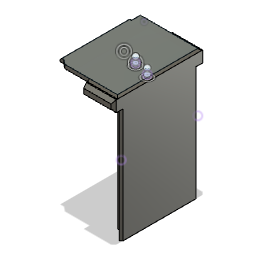
LID (Autodesk Fusion 360 design; units mm, degrees)
Autodesk Fusion 360 part; units mm, degrees
(part 1 of 2)
sketch "Sketch1" plane through (0, 0, 0) normal (0, 1, 0) x (1, 0, 0)
  line L0 (0, 0) -> (18.5, 0)
  line L1 (18.5, 0) -> (18.5, -27.5)
  line L2 (18.5, -27.5) -> (0, -27.5)
  line L3 (0, -27.5) -> (0, 0)
  circle A0 centre (18.5, 0) radius 0.625
  circle A1 centre (0, 0) radius 0.625
  circle A2 centre (0, -27.5) radius 0.625
  circle A3 centre (18.5, -27.5) radius 0.625
  line L4 (-2, -29.5) -> (-2, 2)
  line L5 (-2, 2) -> (20.5, 2)
  line L6 (20.5, 2) -> (20.5, -29.5)
  line L7 (20.5, -29.5) -> (-2, -29.5)
  dimension "d1" = 18.5
  dimension "d2" = 27.5
  dimension "d3" = 1.25
  dimension "d4" = 1.25
  dimension "d5" = 1.25
  dimension "d6" = 1.25
  dimension "d7" = -2
  constraint horizontal L0
  constraint vertical L1
  constraint horizontal L2
  constraint vertical L3
  constraint coincident L0.start L3.end
  constraint coincident L0.end L1.start
  constraint coincident L2.end L3.start
  constraint coincident L1.end L2.start
  measures "d1" distance of L0.start L0.end
  measures "d2" distance of L0.start L2.end
  measures "d3" diameter of A0
  measures "d4" diameter of A1
  measures "d5" diameter of A2
  measures "d6" diameter of A3
sketch "Sketch2" plane through (0, 0, 0) normal (0, -1, 0) x (1, 0, 0)
  circle A0 centre (18.5, 27.5) radius 0.625
  circle A1 centre (18.5, 0) radius 0.625
  circle A2 centre (0, 27.5) radius 0.625
  circle A3 centre (0, 0) radius 0.625
  line L0 (20.5, -2) -> (20.5, 29.5)
  line L1 (20.5, 29.5) -> (-2, 29.5)
  line L2 (-2, 29.5) -> (-2, -2)
  line L3 (-2, -2) -> (20.5, -2)
  line L4 (20.5, 29.5) -> (9.25, 29.5)
  line L5 (9.25, 29.5) -> (9.25, 13.75)
  line L6 (9.25, 13.75) -> (20.5, 13.75)
  line L7 (20.5, 13.75) -> (20.5, 29.5)
  circle A4 centre (9.25, 13.75) radius 4.3
  dimension "d10" = 11.25
  dimension "d11" = 15.75
  dimension "d12" = 8.6
  constraint horizontal L4
  constraint vertical L5
  constraint horizontal L6
  constraint vertical L7
  constraint coincident L0.end L1.start
  constraint coincident L5.end L6.start
  measures "d10" distance of L0.end L4.end
  measures "d11" distance of L0.end L6.end
  measures "d12" diameter of A4
sketch "Sketch3" plane through (0, 3, 0) normal (0, 1, 0) x (-1, 0, 0)
  circle A0 centre (-9.25, 13.75) radius 4.3
  circle A1 centre (-18.5, 27.5) radius 0.625
  circle A2 centre (-18.5, 0) radius 0.625
  circle A3 centre (0, 27.5) radius 0.625
  circle A4 centre (0, 0) radius 0.625
  line L0 (-20.5, 29.5) -> (-20.5, -2)
  line L1 (-20.5, -2) -> (2, -2)
  line L2 (2, -2) -> (2, 29.5)
  line L3 (2, 29.5) -> (-20.5, 29.5)
  line L4 (-15.4346, 2.2358) -> (-15.4346, 25.68) construction
  line L5 (-15.4346, 25.68) -> (-19.6447, 25.68) construction
  line L6 (-19.6447, 25.68) -> (-19.6447, 2.2358) construction
  line L7 (-19.6447, 2.2358) -> (-15.4346, 2.2358) construction
  line L8 (-1.4263, -7.8741) -> (1.1046, 16.1483) construction
  line L9 (1.1046, 16.1483) -> (-2.8567, 16.5657) construction
  line L10 (-2.8567, 16.5657) -> (-5.3876, -7.4567) construction
  line L11 (-5.3876, -7.4567) -> (-1.4263, -7.8741) construction
sketch "Sketch4" plane through (0, 0, 0) normal (0, 1, 0) x (1, 0, 0)
  line L0 (0, 0) -> (122.2, 0)
  line L1 (122.2, 0) -> (122.2, -193)
  line L2 (122.2, -193) -> (0, -193)
  line L3 (0, -193) -> (0, 0)
  dimension "d17" = 122.2
  dimension "d18" = 193
  constraint horizontal L0
  constraint vertical L1
  constraint horizontal L2
  constraint vertical L3
  constraint coincident L0.start L3.end
  measures "d17" distance of L0.start L0.end
  measures "d18" distance of L0.start L2.end
extrude "Extrude4" add sketch "Sketch4" along normal blind 5 makes body 1
extrude "Extrude5" cut 1 faces at (40.7333, 5, 64.3333) along direction (0, -1, 0) blind 5 on bodies 1 bodies 1
sketch "Sketch5" plane through (0, 0, 0) normal (0, 1, 0) x (1, 0, 0)
  line L0 (0, 0) -> (122.2, 0)
  line L1 (122.2, 0) -> (122.2, -193)
  line L2 (122.2, -193) -> (0, -193)
  line L3 (0, -193) -> (0, 0)
  dimension "d23" = 122.2
  dimension "d24" = 193
  constraint horizontal L0
  constraint vertical L1
  constraint horizontal L2
  constraint vertical L3
  constraint coincident L0.start L3.end
  measures "d23" distance of L0.start L0.end
  measures "d24" distance of L0.start L2.end
extrude "Extrude6" add sketch "Sketch5" along normal blind 5 bodies 1
sketch "Sketch6" plane through (0, 5, 0) normal (0, 1, 0) x (-1, 0, 0)
  line L0 (0, 193) -> (-122.2, 193)
  line L1 (-122.2, 193) -> (-122.2, 0)
  line L2 (-122.2, 0) -> (0, 0)
  line L3 (0, 0) -> (0, 193)
  line L4 (0, 193) -> (-10, 193)
  line L5 (-10, 193) -> (-10, 158)
  line L6 (-10, 158) -> (0, 158)
  line L7 (0, 158) -> (0, 193)
  line L8 (0, 0) -> (-10, 0)
  line L9 (-10, 0) -> (-10, 35)
  line L10 (-10, 35) -> (0, 35)
  line L11 (0, 35) -> (0, 0)
  line L12 (-10, 158) -> (-60, 158)
  line L13 (-60, 158) -> (-60, 35)
  line L14 (-60, 35) -> (-10, 35)
  line L15 (-10, 35) -> (-10, 158)
  dimension "d27" = 10
  dimension "d28" = 35
  dimension "d29" = 10
  dimension "d30" = 35
  dimension "d31" = 50
  constraint horizontal L4
  constraint vertical L5
  constraint horizontal L6
  constraint vertical L7
  constraint coincident L0.start L3.end
  constraint horizontal L8
  constraint vertical L9
  constraint horizontal L10
  constraint vertical L11
  constraint coincident L2.end L3.start
  constraint horizontal L12
  constraint vertical L13
  constraint horizontal L14
  constraint vertical L15
  measures "d27" distance of L0.start L4.end
  measures "d28" distance of L0.start L6.end
  measures "d29" distance of L2.end L8.end
  measures "d30" distance of L2.end L10.end
  measures "d31" distance of L5.end L12.end
extrude "Extrude7" cut sketch "Sketch6" against normal blind 5 contours L12 L13 L14 L15 bodies 1
sketch "Sketch7" plane through (0, 5, 0) normal (0, 1, 0) x (-1, 0, 0)
  line L0 (-60, 158) -> (-10, 158)
  line L1 (-10, 158) -> (-10, 35)
  line L2 (-10, 35) -> (-60, 35)
  line L3 (-60, 35) -> (-60, 158)
  line L4 (0, 193) -> (-122.2, 193)
  line L5 (-122.2, 193) -> (-122.2, 0)
  line L6 (-122.2, 0) -> (0, 0)
  line L7 (0, 0) -> (0, 193)
  line L8 (-122.2, 193) -> (-105.075, 193)
  line L9 (-105.075, 193) -> (-105.075, 102)
  line L10 (-105.075, 102) -> (-122.2, 102)
  line L11 (-122.2, 102) -> (-122.2, 193)
  circle A0 centre (-105.075, 102) radius 4
  dimension "d34" = 17.125
  dimension "d35" = 91
  dimension "d36" = 8
  constraint horizontal L8
  constraint vertical L9
  constraint horizontal L10
  constraint vertical L11
  constraint coincident L4.end L5.start
  constraint coincident L9.end L10.start
  measures "d34" distance of L4.end L8.end
  measures "d35" distance of L4.end L10.end
  measures "d36" diameter of A0
extrude "Extrude8" cut sketch "Sketch7" against normal blind 5 contours L9 L10 A0 | L9 L10 A0 bodies 1
sketch "Sketch8" plane through (0, 5, 0) normal (0, 1, 0) x (-1, 0, 0)
  circle A0 centre (-105.075, 102) radius 4
  line L0 (-60, 158) -> (-10, 158)
  line L1 (-10, 158) -> (-10, 35)
  line L2 (-10, 35) -> (-60, 35)
  line L3 (-60, 35) -> (-60, 158)
  line L4 (0, 193) -> (-122.2, 193)
  line L5 (-122.2, 193) -> (-122.2, 0)
  line L6 (-122.2, 0) -> (0, 0)
  line L7 (0, 0) -> (0, 193)
  line L8 (-105.075, 102) -> (-63.325, 102)
  line L9 (-63.325, 102) -> (-63.325, 91)
  line L10 (-63.325, 91) -> (-105.075, 91)
  line L11 (-105.075, 91) -> (-105.075, 102)
  line L12 (-60, 158, -5) -> (-52, 158, -5)
  line L13 (-52, 158, -5) -> (-52, 35, -5)
  line L14 (-52, 35, -5) -> (-60, 35, -5)
  line L15 (-60, 35, -5) -> (-60, 158, -5)
  circle A1 centre (-63.325, 91) radius 4
  point P0 (-60, 158)
  dimension "d39" = 41.75
  dimension "d40" = 11
  dimension "d41" = 8
  dimension "d42" = 8
  constraint horizontal L8
  constraint vertical L9
  constraint horizontal L10
  constraint vertical L11
  constraint coincident A0.centre L8.start
  constraint coincident P0 L0.start
  constraint coincident L9.end L10.start
  measures "d39" distance of A0.centre L8.end
  measures "d40" distance of A0.centre L10.end
  measures "d42" diameter of A1
extrude "Extrude9" add sketch "Sketch8" along normal blind 5 contours L12 L13 L14 L15 in plane through (0, 0, 0) normal (0, 1, 0) bodies 1
sketch "Sketch9" plane through (0, 5, 0) normal (0, 1, 0) x (-1, 0, 0)
  circle A0 centre (-105.075, 102) radius 4
  line L0 (-52, 158) -> (-10, 158)
  line L1 (-10, 158) -> (-10, 35)
  line L2 (-10, 35) -> (-52, 35)
  line L3 (-52, 35) -> (-52, 158)
  line L4 (0, 193) -> (-122.2, 193)
  line L5 (-122.2, 193) -> (-122.2, 0)
  line L6 (-122.2, 0) -> (0, 0)
  line L7 (0, 0) -> (0, 193)
  line L8 (-105.075, 102) -> (-63.325, 102)
  line L9 (-63.325, 102) -> (-63.325, 91)
  line L10 (-63.325, 91) -> (-105.075, 91)
  line L11 (-105.075, 91) -> (-105.075, 102)
  circle A1 centre (-63.325, 91) radius 4
  dimension "d45" = 41.75
  dimension "d46" = 11
  dimension "d47" = 8
  constraint horizontal L8
  constraint vertical L9
  constraint horizontal L10
  constraint vertical L11
  constraint coincident A0.centre L8.start
  constraint coincident L9.end L10.start
  measures "d45" distance of A0.centre L8.end
  measures "d46" distance of A0.centre L10.end
  measures "d47" diameter of A1
extrude "Extrude10" cut sketch "Sketch9" against normal blind 5 contours L9 L10 A1 | L9 L10 A1 bodies 1
sketch "Sketch10" plane through (0, 5, 0) normal (0, 1, 0) x (-1, 0, 0)
  circle A0 centre (-63.325, 91) radius 4
  circle A1 centre (-105.075, 102) radius 4
  line L0 (-52, 158) -> (-10, 158)
  line L1 (-10, 158) -> (-10, 35)
  line L2 (-10, 35) -> (-52, 35)
  line L3 (-52, 35) -> (-52, 158)
  line L4 (0, 193) -> (-122.2, 193)
  line L5 (-122.2, 193) -> (-122.2, 0)
  line L6 (-122.2, 0) -> (0, 0)
  line L7 (0, 0) -> (0, 193)
  line L8 (-122.2, 0) -> (-117.2, 0)
  line L9 (-117.2, 0) -> (-117.2, 2)
  line L10 (-117.2, 2) -> (-122.2, 2)
  line L11 (-122.2, 2) -> (-122.2, 0)
  line L12 (-117.2, 2) -> (-31.2, 2)
  line L13 (-31.2, 2) -> (-31.2, 26)
  line L14 (-31.2, 26) -> (-117.2, 26)
  line L15 (-117.2, 26) -> (-117.2, 2)
  dimension "d50" = 5
  dimension "d51" = 2
  dimension "d52" = 86
  dimension "d53" = 24
  constraint horizontal L8
  constraint vertical L9
  constraint horizontal L10
  constraint vertical L11
  constraint coincident L5.end L6.start
  constraint horizontal L12
  constraint vertical L13
  constraint horizontal L14
  constraint vertical L15
  measures "d50" distance of L5.end L8.end
  measures "d51" distance of L5.end L10.end
  measures "d52" distance of L9.end L12.end
  measures "d53" distance of L9.end L14.end
extrude "Extrude11" cut sketch "Sketch10" against normal blind 5 contours L12 L13 L14 L15 bodies 1
sketch "Sketch11" plane through (0, 5, 0) normal (0, 1, 0) x (-1, 0, 0)
  line L0 (-31.2, 2) -> (-117.2, 2)
  line L1 (-117.2, 2) -> (-117.2, 26)
  line L2 (-117.2, 26) -> (-31.2, 26)
  line L3 (-31.2, 26) -> (-31.2, 2)
  circle A0 centre (-63.325, 91) radius 4
  circle A1 centre (-105.075, 102) radius 4
  line L4 (-52, 158) -> (-10, 158)
  line L5 (-10, 158) -> (-10, 35)
  line L6 (-10, 35) -> (-52, 35)
  line L7 (-52, 35) -> (-52, 158)
  line L8 (0, 193) -> (-122.2, 193)
  line L9 (-122.2, 193) -> (-122.2, 0)
  line L10 (-122.2, 0) -> (0, 0)
  line L11 (0, 0) -> (0, 193)
  line L12 (-122.2, 0) -> (5, 0)
  line L13 (5, 0) -> (5, -5)
  line L14 (5, -5) -> (-122.2, -5)
  line L15 (-122.2, -5) -> (-122.2, 0)
  line L16 (-122.2, 193) -> (5, 193)
  line L17 (5, 193) -> (5, 198)
  line L18 (5, 198) -> (-122.2, 198)
  line L19 (-122.2, 198) -> (-122.2, 193)
  line L20 (5, 193) -> (0, 193)
  line L21 (0, 193) -> (0, 0)
  line L22 (0, 0) -> (5, 0)
  line L23 (5, 0) -> (5, 193)
  dimension "d56" = 127.2
  dimension "d57" = 5
  dimension "d58" = 127.2
  dimension "d59" = 5
  constraint horizontal L12
  constraint vertical L13
  constraint horizontal L14
  constraint vertical L15
  constraint coincident L9.end L10.start
  constraint horizontal L16
  constraint vertical L17
  constraint horizontal L18
  constraint vertical L19
  constraint coincident L8.end L9.start
  constraint horizontal L20
  constraint vertical L21
  constraint horizontal L22
  constraint vertical L23
  constraint coincident L10.end L11.start
  measures "d56" distance of L9.end L12.end
  measures "d57" distance of L9.end L14.end
  measures "d58" distance of L8.end L16.end
  measures "d59" distance of L8.end L18.end
extrude "Extrude12" add sketch "Sketch11" along normal blind 5 bodies 1
sketch "Sketch12" plane through (0, 10, 0) normal (0, 1, 0) x (-1, 0, 0)
  line L0 (-117.2, 26) -> (-31.2, 26)
  line L1 (-31.2, 26) -> (-31.2, 2)
  line L2 (-31.2, 2) -> (-117.2, 2)
  line L3 (-117.2, 2) -> (-117.2, 26)
  circle A0 centre (-105.075, 102) radius 4
  line L4 (-10, 35) -> (-52, 35)
  line L5 (-52, 35) -> (-52, 158)
  line L6 (-52, 158) -> (-10, 158)
  line L7 (-10, 158) -> (-10, 35)
  circle A1 centre (-63.325, 91) radius 4
  line L8 (5, -5) -> (5, 198)
  line L9 (5, 198) -> (-122.2, 198)
  line L10 (-122.2, 198) -> (-122.2, -5)
  line L11 (-122.2, -5) -> (5, -5)
  line L12 (5, 198) -> (10, 198)
  line L13 (10, 198) -> (10, -5)
  line L14 (10, -5) -> (5, -5)
  line L15 (5, -5) -> (5, 198)
  dimension "d62" = 5
  constraint horizontal L12
  constraint vertical L13
  constraint horizontal L14
  constraint vertical L15
  constraint coincident L8.end L9.start
  measures "d62" distance of L8.end L12.end
extrude "Extrude13" add sketch "Sketch12" against normal blind 10 contours L8 L12 L13 L14 L15 bodies 1
extrude "Extrude14" add 1 faces at (-6.6667, 0, 130.3333) along direction (0, -1, 0) blind 45 on bodies 1 bodies 1
extrude "Extrude15" cut 1 faces at (-6.6667, -45, 130.3333) along direction (0, 1, 0) blind 5 on bodies 1 bodies 1
sketch "Sketch13" plane through (0, 10, 0) normal (0, 1, 0) x (-1, 0, 0)
  line L0 (-117.2, 26) -> (-31.2, 26)
  line L1 (-31.2, 26) -> (-31.2, 2)
  line L2 (-31.2, 2) -> (-117.2, 2)
  line L3 (-117.2, 2) -> (-117.2, 26)
  circle A0 centre (-105.075, 102) radius 4
  line L4 (-10, 35) -> (-52, 35)
  line L5 (-52, 35) -> (-52, 158)
  line L6 (-52, 158) -> (-10, 158)
  line L7 (-10, 158) -> (-10, 35)
  circle A1 centre (-63.325, 91) radius 4
  line L8 (10, 198) -> (-122.2, 198)
  line L9 (-122.2, 198) -> (-122.2, -5)
  line L10 (-122.2, -5) -> (10, -5)
  line L11 (10, -5) -> (10, 198)
  line L12 (10, 198) -> (5, 198)
  line L13 (5, 198) -> (5, -5)
  line L14 (5, -5) -> (10, -5)
  line L15 (10, -5) -> (10, 198)
  dimension "d69" = 5
  constraint horizontal L12
  constraint vertical L13
  constraint horizontal L14
  constraint vertical L15
  constraint coincident L8.start L11.end
  measures "d69" distance of L8.start L12.end
extrude "Extrude16" add sketch "Sketch13" along normal blind 30 contours L8 L10 L11 L12 L13 L14 L15 bodies 1
extrude "Extrude17" add 1 faces at (38, 6.6667, 35) along direction (0, 0, 1) blind 12.5 on bodies 1 bodies 1
extrude "Extrude18" add 1 faces at (10, 3.3333, 121.1667) along direction (1, 0, 0) blind 16 on bodies 1 bodies 1
extrude "Extrude19" add 1 faces at (43.3333, 3.3333, 158) along direction (0, 0, -1) blind 7 on bodies 1 bodies 1
extrude "Extrude20" cut 1 faces at (-8.3333, 40, 62.6667) along direction (0, -1, 0) blind 80 on bodies 1 bodies 1
extrude "Extrude21" add 1 faces at (31.2, 3.3333, 18) along direction (1, 0, 0) blind 5 on bodies 1 bodies 1
extrude "Extrude22" cut 1 faces at (90.2, 6.6667, 26) along direction (0, 0, 1) blind 21 on bodies 1 bodies 1
sketch "Sketch14" plane through (0, 10, 0) normal (0, 1, 0) x (-1, 0, 0)
  line L0 (-36.2, 47) -> (-36.2, 2)
  line L1 (-36.2, 2) -> (-117.2, 2)
  line L2 (-117.2, 2) -> (-117.2, 47)
  line L3 (-117.2, 47) -> (-36.2, 47)
  line L4 (5, -5) -> (5, 198)
  line L5 (5, 198) -> (-122.2, 198)
  line L6 (-122.2, 198) -> (-122.2, -5)
  line L7 (-122.2, -5) -> (5, -5)
  circle A0 centre (-105.075, 102) radius 4
  line L8 (-26, 47.5) -> (-52, 47.5)
  line L9 (-52, 47.5) -> (-52, 151)
  line L10 (-52, 151) -> (-26, 151)
  line L11 (-26, 151) -> (-26, 47.5)
  circle A1 centre (-63.325, 91) radius 4
  line L12 (-117.2, 47) -> (-67.2, 47)
  line L13 (-67.2, 47) -> (-67.2, 2)
  line L14 (-67.2, 2) -> (-117.2, 2)
  line L15 (-117.2, 2) -> (-117.2, 47)
  line L16 (-67.2, 47) -> (-36.2, 47)
  line L17 (-36.2, 47, 0) -> (-36.2, 47, -10)
  line L18 (-36.2, 47, -10) -> (-67.2, 47, -10)
  line L19 (-67.2, 47, -10) -> (-67.2, 47, 0)
  point P0 (-36.2, 47)
  dimension "d84" = 50
  constraint horizontal L12
  constraint vertical L13
  constraint horizontal L14
  constraint vertical L15
  constraint coincident L2.end L3.start
  constraint horizontal L16
  constraint coincident P0 L0.start
  measures "d84" distance of L2.end L12.end
extrude "Extrude23" add sketch "Sketch14" against normal blind 5 contours L3 L16 L17 L18 L19 in plane through (0, 10, 47) normal (0, 0, 1) bodies 1
extrude "Extrude24" cut 1 faces at (92.992, 10, 151.6629) along direction (0, -1, 0) blind 5 on bodies 1 bodies 1
sketch "Sketch15" plane through (0, 0, 0) normal (0, -1, 0) x (1, 0, 0)
  line L0 (117.2, 47) -> (117.2, 2)
  line L1 (117.2, 2) -> (36.2, 2)
  line L2 (36.2, 2) -> (36.2, 42)
  line L3 (36.2, 42) -> (67.2, 42)
  line L4 (67.2, 42) -> (67.2, 47)
  line L5 (67.2, 47) -> (117.2, 47)
  circle A0 centre (63.325, 91) radius 4
  circle A1 centre (105.075, 102) radius 4
  line L6 (52, 151) -> (52, 47.5)
  line L7 (52, 47.5) -> (26, 47.5)
  line L8 (26, 47.5) -> (26, 151)
  line L9 (26, 151) -> (52, 151)
  line L10 (122.2, 193) -> (0, 193)
  line L11 (0, 193) -> (0, 0)
  line L12 (0, 0) -> (122.2, 0)
  line L13 (122.2, 0) -> (122.2, 193)
  line L14 (122.2, 193) -> (117.2, 193)
  line L15 (117.2, 193) -> (117.2, 0)
  line L16 (117.2, 0) -> (122.2, 0)
  line L17 (122.2, 0) -> (122.2, 193)
  constraint horizontal L14
  constraint vertical L15
  constraint horizontal L16
  constraint vertical L17
  constraint coincident L12 L15.end
  constraint coincident L10.start L13.end
extrude "Extrude25" add sketch "Sketch15" along normal blind 10 contours L0 L10 L12 L13 L14 L15 L16 L17 bodies 1
extrude "Extrude26" add 1 faces at (118.8667, -10, 128.6667) along direction (0, -1, 0) blind 120 on bodies 1 bodies 1
sketch "Sketch16" plane through (122.2, 0, 0) normal (1, 0, 0) x (0, 0, -1)
  line L0 (0, 5) -> (-193, 5)
  line L1 (-193, 5) -> (-193, -130)
  line L2 (-193, -130) -> (0, -130)
  line L3 (0, -130) -> (0, 5)
  line L4 (-193, 5) -> (-198, 5)
  line L5 (-198, 5) -> (-198, -135)
  line L6 (-198, -135) -> (-193, -135)
  line L7 (-193, -135) -> (-193, 5)
  line L8 (0, 5) -> (5, 5)
  line L9 (5, 5) -> (5, -135)
  line L10 (5, -135) -> (0, -135)
  line L11 (0, -135) -> (0, 5)
  line L12 (-193, -135) -> (0, -135)
  line L13 (0, -135) -> (0, -130)
  line L14 (0, -130) -> (-193, -130)
  line L15 (-193, -130) -> (-193, -135)
  dimension "d93" = 5
  dimension "d94" = 140
  dimension "d95" = 5
  dimension "d96" = 140
  constraint horizontal L4
  constraint vertical L5
  constraint horizontal L6
  constraint vertical L7
  constraint coincident L0.end L1.start
  constraint horizontal L8
  constraint vertical L9
  constraint horizontal L10
  constraint vertical L11
  constraint coincident L0.start L3.end
  constraint horizontal L12
  constraint vertical L13
  constraint horizontal L14
  constraint vertical L15
  constraint coincident L2.end L3.start
  measures "d93" distance of L0.end L4.end
  measures "d94" distance of L0.end L6.end
  measures "d95" distance of L0.start L8.end
  measures "d96" distance of L0.start L10.end
extrude "Extrude27" add sketch "Sketch16" along normal blind 5 bodies 1
sketch "Sketch17" plane through (117.2, 0, 0) normal (-1, 0, 0) x (0, 0, 1)
  line L0 (47, 5) -> (2, 5)
  line L1 (2, 5) -> (2, 0)
  line L2 (2, 0) -> (0, 0)
  line L3 (0, 0) -> (0, -130)
  line L4 (0, -130) -> (193, -130)
  line L5 (193, -130) -> (193, 0)
  line L6 (193, 0) -> (47, 0)
  line L7 (47, 0) -> (47, 5)
  line L8 (185.6716, -122.6716) -> (185.6716, -7.3284)
  line L9 (185.6716, -7.3284) -> (39.6716, -7.3284)
  line L10 (39.6716, -7.3284) -> (39.6716, -2.3284)
  line L11 (39.6716, -2.3284) -> (9.3284, -2.3284)
  line L12 (9.3284, -2.3284) -> (9.3284, -7.3284)
  line L13 (9.3284, -7.3284) -> (7.3284, -7.3284)
  line L14 (7.3284, -7.3284) -> (7.3284, -122.6716)
  line L15 (7.3284, -122.6716) -> (185.6716, -122.6716)
  dimension "d99" = -7.3284
extrude "Extrude28" cut sketch "Sketch17" against normal blind 5 contours L8 L9 L10 L11 L12 L13 L14 L15 bodies 1
extrude "Extrude29" cut 1 faces at (36.2, 3.3333, 15.3333) along direction (-1, 0, 0) blind 2 on bodies 1 bodies 1
extrude "Extrude30" add 1 faces at (52, 1.6667, 82) along direction (-1, 0, 0) blind 5 on bodies 1 bodies 1
extrude "Extrude31" add 1 faces at (40, 1.6667, 151) along direction (0, 0, -1) blind 2 on bodies 1 bodies 1
sketch "Sketch18" plane through (0, 5, 0) normal (0, 1, 0) x (-1, 0, 0)
  circle A0 centre (-63.325, 91) radius 4
  line L0 (-26, 149) -> (-26, 47.5)
  line L1 (-26, 47.5) -> (-47, 47.5)
  line L2 (-47, 47.5) -> (-47, 149)
  line L3 (-47, 149) -> (-26, 149)
  circle A1 centre (-105.075, 102) radius 4
  line L4 (-67.2, 42) -> (-34.2, 42)
  line L5 (-34.2, 42) -> (-34.2, 2)
  line L6 (-34.2, 2) -> (-117.2, 2)
  line L7 (-117.2, 2) -> (-117.2, 47)
  line L8 (-117.2, 47) -> (-67.2, 47)
  line L9 (-67.2, 47) -> (-67.2, 42)
  line L10 (-122.2, 0) -> (0, 0)
  line L11 (0, 0) -> (0, 193)
  line L12 (0, 193) -> (-122.2, 193)
  line L13 (-122.2, 193) -> (-122.2, 198)
  line L14 (-122.2, 198) -> (-127.2, 198)
  line L15 (-127.2, 198) -> (-127.2, -5)
  line L16 (-127.2, -5) -> (-122.2, -5)
  line L17 (-122.2, -5) -> (-122.2, 0)
  line L18 (-119.2, 0) -> (-119.2, 49)
  line L19 (-119.2, 49) -> (-65.2, 49)
  line L20 (-65.2, 49) -> (-65.2, 44)
  line L21 (-65.2, 44) -> (-32.2, 44)
  line L22 (-32.2, 44) -> (-32.2, 0)
  line L23 (-32.2, 0) -> (-119.2, 0)
  dimension "d108" = -2
extrude "Extrude32" add sketch "Sketch18" along normal blind 5 contours L10 L18 L19 L20 L21 L22 L23 bodies 1
sketch "Sketch19" plane through (0, 5, 0) normal (0, 1, 0) x (-1, 0, 0)
  line L0 (-119.2, 0) -> (-119.2, 49)
  line L1 (-119.2, 49) -> (-65.2, 49)
  line L2 (-65.2, 49) -> (-65.2, 44)
  line L3 (-65.2, 44) -> (-32.2, 44)
  line L4 (-32.2, 44) -> (-32.2, 0)
  line L5 (-32.2, 0) -> (0, 0)
  line L6 (0, 0) -> (0, 193)
  line L7 (0, 193) -> (-122.2, 193)
  line L8 (-122.2, 193) -> (-122.2, 198)
  line L9 (-122.2, 198) -> (-127.2, 198)
  line L10 (-127.2, 198) -> (-127.2, -5)
  line L11 (-127.2, -5) -> (-122.2, -5)
  line L12 (-122.2, -5) -> (-122.2, 0)
  line L13 (-122.2, 0) -> (-119.2, 0)
  circle A0 centre (-105.075, 102) radius 4
  line L14 (-26, 149) -> (-26, 47.5)
  line L15 (-26, 47.5) -> (-47, 47.5)
  line L16 (-47, 47.5) -> (-47, 149)
  line L17 (-47, 149) -> (-26, 149)
  circle A1 centre (-63.325, 91) radius 4
  line L18 (-49, 45.5) -> (-49, 151)
  line L19 (-49, 151) -> (-24, 151)
  line L20 (-24, 151) -> (-24, 45.5)
  line L21 (-24, 45.5) -> (-49, 45.5)
  dimension "d111" = -2
extrude "Extrude33" add sketch "Sketch19" along normal blind 5 contours L18 L19 L20 L21 bodies 1
extrude "Extrude34" add 1 faces at (122.2, -84.2239, 77.5572) along direction (-1, 0, 0) blind 5 on bodies 1 bodies 1
sketch "Sketch20" plane through (127.2, 0, 0) normal (1, 0, 0) x (0, 0, -1)
  line L0 (-198, -135) -> (5, -135)
extrude "Extrude35" cut 1 faces at (61.8667, 10, 0.6667) along direction (0, -1, 0) blind 5 on bodies 1 bodies 1
extrude "Extrude36" cut 1 faces at (48.3333, 10, 81.3333) along direction (0, -1, 0) blind 5 on bodies 1 bodies 1
sketch "Sketch21" plane through (0, 5, 0) normal (0, 1, 0) x (-1, 0, 0)
  line L0 (-47, 47.5) -> (-47, 149)
  line L1 (-47, 149) -> (-26, 149)
  line L2 (-26, 149) -> (-26, 47.5)
  line L3 (-26, 47.5) -> (-47, 47.5)
  line L4 (-117.2, 47) -> (-67.2, 47)
  line L5 (-67.2, 47) -> (-67.2, 42)
  line L6 (-67.2, 42) -> (-34.2, 42)
  line L7 (-34.2, 42) -> (-34.2, 2)
  line L8 (-34.2, 2) -> (-117.2, 2)
  line L9 (-117.2, 2) -> (-117.2, 47)
  line L10 (-122.2, 0) -> (0, 0)
  line L11 (0, 0) -> (0, 193)
  line L12 (0, 193) -> (-122.2, 193)
  line L13 (-122.2, 193) -> (-122.2, 198)
  line L14 (-122.2, 198) -> (-127.2, 198)
  line L15 (-127.2, 198) -> (-127.2, -5)
  line L16 (-127.2, -5) -> (-122.2, -5)
  line L17 (-122.2, -5) -> (-122.2, 0)
  circle A0 centre (-105.075, 102) radius 4
  circle A1 centre (-63.325, 91) radius 4
  line L18 (0, 193) -> (-10, 193)
  line L19 (-10, 193) -> (-10, 183)
  line L20 (-10, 183) -> (0, 183)
  line L21 (0, 183) -> (0, 193)
  line L22 (0, 0) -> (-10, 0)
  line L23 (-10, 0) -> (-10, 10)
  line L24 (-10, 10) -> (0, 10)
  line L25 (0, 10) -> (0, 0)
  circle A2 centre (-10, 183) radius 4
  circle A3 centre (-10, 10) radius 4
  dimension "d120" = 10
  dimension "d121" = 10
  dimension "d122" = 10
  dimension "d123" = 10
  dimension "d124" = 8
  dimension "d125" = 8
  constraint horizontal L18
  constraint vertical L19
  constraint horizontal L20
  constraint vertical L21
  constraint coincident L11.end L12.start
  constraint horizontal L22
  constraint vertical L23
  constraint horizontal L24
  constraint vertical L25
  constraint coincident L10.end L11.start
  constraint coincident L19.end L20.start
  constraint coincident L23.end L24.start
  measures "d120" distance of L11.end L18.end
  measures "d121" distance of L11.end L20.end
  measures "d122" distance of L10.end L22.end
  measures "d123" distance of L10.end L24.end
  measures "d124" diameter of A2
  measures "d125" diameter of A3
extrude "Extrude37" cut sketch "Sketch21" against normal blind 5 contours L23 L24 A3 | L23 L24 A3 | L19 L20 A2 | L19 L20 A2 bodies 1
fillet "Fillet1" radius 5 1 edges at (127.2, -65, -5) on bodies 1
fillet "Fillet2" radius 5 1 edges at (127.2, -65, 198) on bodies 1
fillet "Fillet3" radius 5 3 edges at (125.7355, -135, 196.5355) (127.2, -135, 96.5) (125.7355, -135, -3.5355) on bodies 1
sketch "Sketch22" plane through (127.2, 0, 0) normal (1, 0, 0) x (0, 0, -1)
  line L0 (-163.3282, -18.9561) -> (-150.9282, -18.9561)
  line L1 (-150.9282, -18.9561) -> (-150.9282, -35.9561)
  line L2 (-150.9282, -35.9561) -> (-163.3282, -35.9561)
  line L3 (-163.3282, -35.9561) -> (-163.3282, -18.9561)
  dimension "d134" = 12.4
  dimension "d135" = 17
  constraint horizontal L0
  constraint vertical L1
  constraint horizontal L2
  constraint vertical L3
  measures "d134" distance of L0.start L0.end
  measures "d135" distance of L0.start L2.end
extrude "Extrude38" cut sketch "Sketch22" against normal blind 10 bodies 1
sketch "Sketch23" plane through (117.2, 0, 0) normal (-1, 0, 0) x (0, 0, 1)
  line L0 (150.9282, -35.9561) -> (150.9282, -18.9561)
  line L1 (150.9282, -18.9561) -> (163.3282, -18.9561)
  line L2 (163.3282, -18.9561) -> (163.3282, -35.9561)
  line L3 (163.3282, -35.9561) -> (150.9282, -35.9561)
  line L4 (47, 5) -> (2, 5)
  line L5 (2, 5) -> (2, 0)
  line L6 (2, 0) -> (0, 0)
  line L7 (0, 0) -> (0, -130)
  line L8 (0, -130) -> (193, -130)
  line L9 (193, -130) -> (193, 0)
  line L10 (193, 0) -> (47, 0)
  line L11 (47, 0) -> (47, 5)
  line L12 (168.3282, -40.9561) -> (145.9282, -40.9561)
  line L13 (145.9282, -40.9561) -> (145.9282, -13.9561)
  line L14 (145.9282, -13.9561) -> (168.3282, -13.9561)
  line L15 (168.3282, -13.9561) -> (168.3282, -40.9561)
  dimension "d138" = -5
extrude "Extrude39" cut sketch "Sketch23" against normal blind 6.5 contours L12 L13 L14 L15 bodies 1
extrude "Extrude40" cut 6 faces at (122.2007, -40.0003, 198) (122.2003, -135, 128.667) (122.2007, -40.0003, -5) (122.2, -133.3333, 64.3333) (122.2007, -130.4762, 197.9774) (122.2007, -130.2389, -4.9943) along direction (1, 0, 0) blind 5 on bodies 1 bodies 1
sketch "Sketch24" plane through (0, 0, 0) normal (1, 0, 0) x (0, 0, -1)
  line L0 (-47, 5, 67.2) -> (-42, 5, 67.2)
  line L1 (-42, 5, 67.2) -> (-42, 5, 34.2)
  line L2 (-42, 5, 34.2) -> (-47, 5, 34.2)
  line L3 (-47, 5, 34.2) -> (-47, 5, 67.2)
  point P0 (-47, 5)
  point P1 (-42, 5)
extrude "Extrude41" cut sketch "Sketch24" against normal blind 5 contours L0 L1 L2 L3 in plane through (0, 5, 0) normal (0, 1, 0) bodies 1
sketch "Sketch25" plane through (0, 5, 0) normal (0, 1, 0) x (-1, 0, 0)
  line L0 (-34.2, 47) -> (-34.2, 2)
  line L1 (-34.2, 2) -> (-117.2, 2)
  line L2 (-117.2, 2) -> (-117.2, 47)
  line L3 (-117.2, 47) -> (-34.2, 47)
  circle A0 centre (-63.325, 91) radius 4
  circle A1 centre (-105.075, 102) radius 4
  line L4 (-47, 47.5) -> (-47, 149)
  line L5 (-47, 149) -> (-26, 149)
  line L6 (-26, 149) -> (-26, 47.5)
  line L7 (-26, 47.5) -> (-47, 47.5)
  circle A2 centre (-10, 10) radius 4
  circle A3 centre (-10, 183) radius 4
  line L8 (0, 193) -> (-127.2, 193)
  line L9 (-127.2, 193) -> (-127.2, 0)
  line L10 (-127.2, 0) -> (0, 0)
  line L11 (0, 0) -> (0, 193)
  line L12 (-127.2, 193) -> (-117.2, 193)
  line L13 (-117.2, 193) -> (-117.2, 191)
  line L14 (-117.2, 191) -> (-127.2, 191)
  line L15 (-127.2, 191) -> (-127.2, 193)
  line L16 (-117.2, 191) -> (-34.2, 191)
  line L17 (-34.2, 191) -> (-34.2, 146)
  line L18 (-34.2, 146) -> (-117.2, 146)
  line L19 (-117.2, 146) -> (-117.2, 191)
  dimension "d145" = 10
  dimension "d146" = 2
  dimension "d147" = 83
  dimension "d148" = 45
  constraint horizontal L12
  constraint vertical L13
  constraint horizontal L14
  constraint vertical L15
  constraint coincident L8.end L9.start
  constraint horizontal L16
  constraint vertical L17
  constraint horizontal L18
  constraint vertical L19
  measures "d145" distance of L8.end L12.end
  measures "d146" distance of L8.end L14.end
  measures "d147" distance of L13.end L16.end
  measures "d148" distance of L13.end L18.end
extrude "Extrude42" cut sketch "Sketch25" against normal blind 10 contours L4 L5 L16 L17 L18 L19 bodies 1
sketch "Sketch26" plane through (0, 5, 0) normal (0, 1, 0) x (-1, 0, 0)
  line L0 (0, 193) -> (-127.2, 193)
  line L1 (-127.2, 193) -> (-127.2, 0)
  line L2 (-127.2, 0) -> (0, 0)
  line L3 (0, 0) -> (0, 193)
  circle A0 centre (-10, 183) radius 4
  circle A1 centre (-10, 10) radius 4
  line L4 (-47, 146) -> (-117.2, 146)
  line L5 (-117.2, 146) -> (-117.2, 191)
  line L6 (-117.2, 191) -> (-34.2, 191)
  line L7 (-34.2, 191) -> (-34.2, 149)
  line L8 (-34.2, 149) -> (-26, 149)
  line L9 (-26, 149) -> (-26, 47.5)
  line L10 (-26, 47.5) -> (-47, 47.5)
  line L11 (-47, 47.5) -> (-47, 146)
  circle A2 centre (-105.075, 102) radius 4
  circle A3 centre (-63.325, 91) radius 4
  line L12 (-34.2, 47) -> (-34.2, 2)
  line L13 (-34.2, 2) -> (-117.2, 2)
  line L14 (-117.2, 2) -> (-117.2, 47)
  line L15 (-117.2, 47) -> (-34.2, 47)
  line L16 (-127.2, 193) -> (0, 193)
  line L17 (0, 193) -> (0, 198)
  line L18 (0, 198) -> (-127.2, 198)
  line L19 (-127.2, 198) -> (-127.2, 193)
  line L20 (-127.2, 193) -> (0, 193)
  line L21 (0, 193) -> (0, 191)
  line L22 (0, 191) -> (-127.2, 191)
  line L23 (-127.2, 191) -> (-127.2, 193)
  dimension "d151" = 5
  constraint horizontal L16
  constraint vertical L17
  constraint horizontal L18
  constraint vertical L19
  constraint coincident L0.end L1.start
  constraint horizontal L20
  constraint vertical L21
  constraint horizontal L22
  constraint vertical L23
  constraint coincident L3 L21.end
  measures "d151" distance of L0.end L18.end
extrude "Extrude43" add sketch "Sketch26" along normal blind 5 contours L0 L1 L3 L6 L16 L20 L21 L22 L23 | L0 L16 L17 L18 L19 L20 bodies 1
extrude "Extrude44" cut 1 faces at (84.8, 10, 195.6667) along direction (0, -1, 0) blind 5 on bodies 1 bodies 1
extrude "Extrude45" cut 1 faces at (127.2, -53.652, 50.3094) along direction (-1, 0, 0) blind 10 on bodies 1 bodies 1
extrude "Extrude46" add 1 faces at (89.5333, 3.3333, 2) along direction (0, 0, 1) blind 45 on bodies 1 bodies 1
extrude "Extrude47" add 1 faces at (33, 1.6667, 47.5) along direction (0, 0, 1) blind 98.5 on bodies 1 bodies 1
extrude "Extrude48" add 1 faces at (56.4, 3.3333, 146) along direction (0, 0, 1) blind 3 on bodies 1 bodies 1
extrude "Extrude49" add 1 faces at (61.8667, 1.6667, 149) along direction (0, 0, 1) blind 42 on bodies 1 bodies 1
sketch "Sketch27" plane through (0, 5, 0) normal (0, 1, 0) x (-1, 0, 0)
  line L0 (-117.2, 193) -> (-117.2, 0)
  line L1 (-117.2, 0) -> (0, 0)
  line L2 (0, 0) -> (0, 193)
  line L3 (0, 193) -> (-117.2, 193)
  circle A0 centre (-10, 183) radius 4
  circle A1 centre (-10, 10) radius 4
  circle A2 centre (-105.075, 102) radius 4
  circle A3 centre (-63.325, 91) radius 4
  circle A4 centre (-10, 183) radius 4
  circle A5 centre (-10, 10) radius 4
  constraint concentric A0 A4
  constraint concentric A1 A5
extrude "Extrude50" add sketch "Sketch27" against normal blind 5 contours A0 A4 | A1 A5 bodies 1
sketch "Sketch28" plane through (0, 5, 0) normal (0, 1, 0) x (-1, 0, 0)
  line L0 (-117.2, 193) -> (-117.2, 0)
  line L1 (-117.2, 0) -> (0, 0)
  line L2 (0, 0) -> (0, 193)
  line L3 (0, 193) -> (-117.2, 193)
  circle A0 centre (-105.075, 102) radius 4
  circle A1 centre (-63.325, 91) radius 4
extrude "Extrude51" add 1 faces at (117.2, 1.6667, 128.6667) along direction (1, 0, 0) blind 5 on bodies 1 bodies 1
sketch "Sketch29" plane through (0, 0, 0) normal (0, -1, 0) x (1, 0, 0)
  line L0 (122.2, 193) -> (0, 193)
  line L1 (0, 193) -> (0, 0)
  line L2 (0, 0) -> (122.2, 0)
  line L3 (122.2, 0) -> (122.2, 193)
  circle A0 centre (63.325, 91) radius 4
  circle A1 centre (105.075, 102) radius 4
  line L4 (122.2, 193) -> (117.2, 193)
  line L5 (117.2, 193) -> (117.2, 0)
  line L6 (117.2, 0) -> (122.2, 0)
  line L7 (122.2, 0) -> (122.2, 193)
  dimension "d170" = 5
  constraint horizontal L4
  constraint vertical L5
  constraint horizontal L6
  constraint vertical L7
  constraint coincident L0.start L3.end
  measures "d170" distance of L0.start L4.end
extrude "Extrude52" add 1 faces at (81.4667, 3.3333, 193) along direction (0, 0, 1) blind 5 on bodies 1 bodies 1
extrude "Extrude53" add 1 faces at (81.4667, 1.6667, 0) along direction (0, 0, -1) blind 5 on bodies 1 bodies 1
extrude "Extrude54" add sketch "Sketch29" along normal blind 298 contours L0 L2 L3 L4 L5 L6 L7 bodies 1
extrude "Extrude55" add 1 faces at (120.5333, -99.3333, 193) along direction (0, 0, 1) blind 5 on bodies 1 bodies 1
extrude "Extrude56" add 1 faces at (118.8667, -99.3333, 0) along direction (0, 0, -1) blind 5 on bodies 1 bodies 1
extrude "Extrude57" add 1 faces at (0, 3.3333, 62.6667) along direction (-1, 0, 0) blind 15 on bodies 1 bodies 1
sketch "Sketch30" plane through (0, 0, 198) normal (0, 0, 1) x (1, 0, 0)
  line L0 (122.2, 5) -> (-15, 5)
  line L1 (-15, 5) -> (-15, 0)
  line L2 (-15, 0) -> (117.2, 0)
  line L3 (117.2, 0) -> (117.2, -298)
  line L4 (117.2, -298) -> (122.2, -298)
  line L5 (122.2, -298) -> (122.2, 5)
  line L6 (122.2, 5) -> (52.2, 5)
  line L7 (52.2, 5) -> (52.2, 0)
  line L8 (52.2, 0) -> (122.2, 0)
  line L9 (122.2, 0) -> (122.2, 5)
  dimension "d183" = 70
  constraint horizontal L6
  constraint vertical L7
  constraint horizontal L8
  constraint vertical L9
  constraint coincident L0.start L5.end
  measures "d183" distance of L0.start L6.end
extrude "Extrude58" add sketch "Sketch30" along normal blind 5 contours L0 L2 L5 L6 L7 L8 L9 bodies 1
extrude "Extrude59" cut 1 faces at (120.5333, -198.6667, 198) along direction (0, 0, -1) blind 5 on bodies 1 bodies 1
sketch "Sketch31" plane through (0, 0, -5) normal (0, 0, -1) x (-1, 0, 0)
  line L0 (-117.2, 0) -> (15, 0)
  line L1 (15, 0) -> (15, 5)
  line L2 (15, 5) -> (-122.2, 5)
  line L3 (-122.2, 5) -> (-122.2, -298)
  line L4 (-122.2, -298) -> (-117.2, -298)
  line L5 (-117.2, -298) -> (-117.2, 0)
  line L6 (-117.2, 0) -> (-122.2, 0)
  line L7 (-122.2, 0) -> (-122.2, -298)
  line L8 (-122.2, -298) -> (-117.2, -298)
  line L9 (-117.2, -298) -> (-117.2, 0)
  constraint horizontal L6
  constraint vertical L7
  constraint horizontal L8
  constraint vertical L9
  constraint coincident L3.end L4.start
  constraint coincident L0.start L5.end
extrude "Extrude60" cut sketch "Sketch31" against normal blind 5 contours L3 L4 L5 L6 L7 L8 L9 bodies 1
extrude "Extrude61" add 1 faces at (75.5333, 3.3333, 203) along direction (0, 0, 1) blind 15 on bodies 1 bodies 1
sketch "Sketch32" plane through (0, 0, 0) normal (0, -1, 0) x (1, 0, 0)
  circle A0 centre (105.075, 102) radius 4
  circle A1 centre (63.325, 91) radius 4
  line L0 (117.2, 0) -> (117.2, 193)
  line L1 (117.2, 193) -> (122.2, 193)
  line L2 (122.2, 193) -> (122.2, 218)
  line L3 (122.2, 218) -> (52.2, 218)
  line L4 (52.2, 218) -> (52.2, 198)
  line L5 (52.2, 198) -> (-15, 198)
  line L6 (-15, 198) -> (-15, -5)
  line L7 (-15, -5) -> (122.2, -5)
  line L8 (122.2, -5) -> (122.2, 0)
  line L9 (122.2, 0) -> (117.2, 0)
  line L10 (52.2, 218) -> (122.2, 218)
  line L11 (122.2, 218) -> (122.2, 198)
  line L12 (122.2, 198) -> (52.2, 198)
  line L13 (52.2, 198) -> (52.2, 218)
  constraint horizontal L10
  constraint vertical L11
  constraint horizontal L12
  constraint vertical L13
  constraint coincident L2 L11.end
  constraint coincident L3.end L4.start
extrude "Extrude62" add sketch "Sketch32" along normal blind 20 contours L2 L3 L4 L10 L11 L12 L13 bodies 1
extrude "Extrude63" cut 1 faces at (98.8667, -6.6667, 198) along direction (0, 0, 1) blind 0.4 on bodies 1 bodies 1
extrude "Extrude64" add 1 faces at (122.2, -99.3333, 128.6667) along direction (1, 0, 0) blind 5 on bodies 1 bodies 1
extrude "Extrude65" cut 1 faces at (127.2, -99.3333, 128.6667) along direction (-1, 0, 0) blind 5 on bodies 1 bodies 1
extrude "Extrude66" add 1 faces at (117.2, -99.3333, 128.6667) along direction (-1, 0, 0) blind 4.5 on bodies 1 bodies 1
sketch "Sketch33" plane through (0, 0, -5) normal (0, 0, -1) x (-1, 0, 0)
  line L0 (-122.2, 5) -> (-122.2, 0)
  line L1 (-122.2, 0) -> (15, 0)
  line L2 (15, 0) -> (15, 5)
  line L3 (15, 5) -> (-122.2, 5)
  line L4 (-122.2, 5) -> (-46.2, 5)
  line L5 (-46.2, 5) -> (-46.2, 0)
  line L6 (-46.2, 0) -> (-122.2, 0)
  line L7 (-122.2, 0) -> (-122.2, 5)
  dimension "d202" = 76
  constraint horizontal L4
  constraint vertical L5
  constraint horizontal L6
  constraint vertical L7
  constraint coincident L0.start L3.end
  measures "d202" distance of L0.start L4.end
extrude "Extrude67" add sketch "Sketch33" along normal blind 20 contours L0 L1 L3 L4 L5 L6 L7 bodies 1
sketch "Sketch34" plane through (0, 0, 0) normal (0, -1, 0) x (1, 0, 0)
  line L0 (112.7, 193) -> (122.2, 193)
  line L1 (122.2, 193) -> (122.2, 198.4)
  line L2 (122.2, 198.4) -> (52.2, 198.4)
  line L3 (52.2, 198.4) -> (52.2, 198)
  line L4 (52.2, 198) -> (-15, 198)
  line L5 (-15, 198) -> (-15, -5)
  line L6 (-15, -5) -> (46.2, -5)
  line L7 (46.2, -5) -> (46.2, -25)
  line L8 (46.2, -25) -> (122.2, -25)
  line L9 (122.2, -25) -> (122.2, 0)
  line L10 (122.2, 0) -> (112.7, 0)
  line L11 (112.7, 0) -> (112.7, 193)
  circle A0 centre (105.075, 102) radius 4
  circle A1 centre (63.325, 91) radius 4
  line L12 (46.2, -25) -> (122.2, -25)
  line L13 (122.2, -25) -> (122.2, -5.4)
  line L14 (122.2, -5.4) -> (46.2, -5.4)
  line L15 (46.2, -5.4) -> (46.2, -25)
  dimension "d205" = 19.6
  constraint horizontal L12
  constraint vertical L13
  constraint horizontal L14
  constraint vertical L15
  constraint coincident L7.end L8.start
  measures "d205" distance of L7.end L14.end
extrude "Extrude68" add sketch "Sketch34" along normal blind 20 contours L7 L8 L9 L12 L13 L14 L15 bodies 1
extrude "Extrude69" add 1 faces at (52.2, -5, 211.4667) along direction (-1, 0, 0) blind 6 on bodies 1 bodies 1
extrude "Extrude70" cut 1 faces at (46.2, -5, 211.4667) along direction (1, 0, 0) blind 1.5 on bodies 1 bodies 1
extrude "Extrude71" cut 1 faces at (46.2, -5, -18.4667) along direction (1, 0, 0) blind 1.5 on bodies 1 bodies 1
extrude "Extrude72" add 1 faces at (47.7, -5, -18.4667) along direction (-1, 0, 0) blind 1 on bodies 1 bodies 1
sketch "Sketch35" plane through (122.2, 0, 0) normal (1, 0, 0) x (0, 0, -1)
  line L0 (-198.4, -20) -> (-198.4, 0)
  line L1 (-198.4, 0) -> (-193, 0)
  line L2 (-193, 0) -> (-193, -298)
  line L3 (-193, -298) -> (0, -298)
  line L4 (0, -298) -> (0, 0)
  line L5 (0, 0) -> (5.4, 0)
  line L6 (5.4, 0) -> (5.4, -20)
  line L7 (5.4, -20) -> (25, -20)
  line L8 (25, -20) -> (25, 5)
  line L9 (25, 5) -> (-218, 5)
  line L10 (-218, 5) -> (-218, -20)
  line L11 (-218, -20) -> (-198.4, -20)
  line L12 (-198.4, 5) -> (5.4, 5)
  line L13 (5.4, 5) -> (5.4, -298)
  line L14 (5.4, -298) -> (-198.4, -298)
  line L15 (-198.4, -298) -> (-198.4, 5)
  constraint horizontal L12
  constraint vertical L13
  constraint horizontal L14
  constraint vertical L15
  constraint coincident L9 L12.start
extrude "Extrude73" add sketch "Sketch35" along normal blind 5 separate body contours L0 L1 L2 L14 L15 | L1 L2 L3 L4 L5 L9 L12 L13 L14 L15 | L4 L5 L6 L13 L14 makes body 2
sketch "Sketch36" plane through (122.2, 0, 0) normal (1, 0, 0) x (0, 0, -1)
  line L0 (-198.4, -20) -> (-198.4, 0)
  line L1 (-198.4, 0) -> (-193, 0)
  line L2 (-193, 0) -> (-193, -298)
  line L3 (-193, -298) -> (0, -298)
  line L4 (0, -298) -> (0, 0)
  line L5 (0, 0) -> (5.4, 0)
  line L6 (5.4, 0) -> (5.4, -20)
  line L7 (5.4, -20) -> (25, -20)
  line L8 (25, -20) -> (25, 5)
  line L9 (25, 5) -> (-218, 5)
  line L10 (-218, 5) -> (-218, -20)
  line L11 (-218, -20) -> (-198.4, -20)
  line L12 (-198.4, 5) -> (-218, 5)
  line L13 (-218, 5) -> (-218, -20)
  line L14 (-218, -20) -> (-198.4, -20)
  line L15 (-198.4, -20) -> (-198.4, 5)
  line L16 (5.4, 5) -> (25, 5)
  line L17 (25, 5) -> (25, -20)
  line L18 (25, -20) -> (5.4, -20)
  line L19 (5.4, -20) -> (5.4, 5)
  point P0 (-198.4, 5)
  point P1 (5.4, 5)
  constraint horizontal L12
  constraint vertical L13
  constraint horizontal L14
  constraint vertical L15
  constraint coincident L10.end L11.start
  constraint coincident P0 L12.start
  constraint horizontal L16
  constraint vertical L17
  constraint horizontal L18
  constraint vertical L19
  constraint coincident L7.end L8.start
  constraint coincident P1 L16.start
extrude "Extrude74" add sketch "Sketch36" along normal blind 5 contours L0 L9 L10 L11 L12 L13 L14 L15 | L6 L7 L8 L9 L16 L17 L18 L19 bodies 1 2
extrude "Extrude75" add 1 faces at (115.8667, -298, 64.3333) along direction (0, -1, 0) blind 5 on bodies 1 bodies 1
extrude "Extrude76" cut 1 faces at (115.8667, -303, 64.3333) along direction (0, 1, 0) blind 5 on bodies 1 bodies 1
extrude "Extrude77" add 1 faces at (115.8667, -298, 64.3333) along direction (0, -1, 0) blind 5 on bodies 1 bodies 1
sketch "Sketch37" plane through (0, 5, 0) normal (0, 1, 0) x (-1, 0, 0)
  line L0 (-46.7, -5) -> (15, -5)
  line L1 (15, -5) -> (15, 198)
  line L2 (15, 198) -> (-47.7, 198)
  line L3 (-47.7, 198) -> (-47.7, 218)
  line L4 (-47.7, 218) -> (-127.2, 218)
  line L5 (-127.2, 218) -> (-127.2, -25)
  line L6 (-127.2, -25) -> (-46.7, -25)
  line L7 (-46.7, -25) -> (-46.7, -5)
  circle A0 centre (-63.325, 91) radius 4
  circle A1 centre (-105.075, 102) radius 4
  line L8 (-127.2, -25) -> (15, -25)
  line L9 (15, -25) -> (15, 218)
  line L10 (15, 218) -> (-127.2, 218)
  line L11 (-127.2, 218) -> (-127.2, -25)
  constraint horizontal L8
  constraint vertical L9
  constraint horizontal L10
  constraint vertical L11
  constraint coincident L5.end L6.start
extrude "Extrude78" add sketch "Sketch37" along normal blind 5 bodies 1
sketch "Sketch38" plane through (0, 0, -25) normal (0, 0, -1) x (-1, 0, 0)
  line L0 (-127.2, 10) -> (-127.2, -20)
  line L1 (-127.2, -20) -> (-46.7, -20)
  line L2 (-46.7, -20) -> (-46.7, 5)
  line L3 (-46.7, 5) -> (15, 5)
  line L4 (15, 5) -> (15, 10)
  line L5 (15, 10) -> (-127.2, 10)
  line L6 (-46.7, 5) -> (15, 5)
  line L7 (15, 5) -> (15, 10)
  line L8 (15, 10) -> (-46.7, 10)
  line L9 (-46.7, 10) -> (-46.7, 5)
  constraint horizontal L6
  constraint vertical L7
  constraint horizontal L8
  constraint vertical L9
  constraint coincident L4.end L5.start
  constraint coincident L2.end L3.start
extrude "Extrude79" cut sketch "Sketch38" against normal blind 20 contours L3 L4 L5 L6 L7 L8 L9 bodies 1
sketch "Sketch39" plane through (0, 0, 218) normal (0, 0, 1) x (1, 0, 0)
  line L0 (47.7, 5) -> (47.7, -20)
  line L1 (47.7, -20) -> (127.2, -20)
  line L2 (127.2, -20) -> (127.2, 10)
  line L3 (127.2, 10) -> (-15, 10)
  line L4 (-15, 10) -> (-15, 5)
  line L5 (-15, 5) -> (47.7, 5)
  line L6 (47.7, 5) -> (-15, 5)
  line L7 (-15, 5) -> (-15, 10)
  line L8 (-15, 10) -> (47.7, 10)
  line L9 (47.7, 10) -> (47.7, 5)
  constraint horizontal L6
  constraint vertical L7
  constraint horizontal L8
  constraint vertical L9
  constraint coincident L3.end L4.start
  constraint coincident L0.start L5.end
extrude "Extrude80" cut sketch "Sketch39" against normal blind 20 contours L3 L4 L5 L6 L7 L8 L9 bodies 1
extrude "Extrude81" add 1 faces at (5.9, 6.6667, 198) along direction (0, 0, 1) blind 5 on bodies 1 bodies 1
sketch "Sketch40" plane through (0, 0, 203) normal (0, 0, 1) x (1, 0, 0)
  line L0 (-15, 10) -> (-15, 0)
  line L1 (-15, 0) -> (47.7, 0)
  line L2 (47.7, 0) -> (47.7, 10)
  line L3 (47.7, 10) -> (-15, 10)
  line L4 (-15, 10) -> (47.7, 10)
  line L5 (47.7, 10) -> (47.7, 5)
  line L6 (47.7, 5) -> (-15, 5)
  line L7 (-15, 5) -> (-15, 10)
  dimension "d234" = 5
  constraint horizontal L4
  constraint vertical L5
  constraint horizontal L6
  constraint vertical L7
  constraint coincident L2 L5.end
  constraint coincident L0.start L3.end
  measures "d234" distance of L0.start L6.end
extrude "Extrude82" add sketch "Sketch40" along normal blind 5 contours L0 L2 L3 L4 L5 L6 L7 bodies 1
sketch "Sketch41" plane through (0, 0, -5) normal (0, 0, -1) x (-1, 0, 0)
  line L0 (-46.7, 10) -> (-46.7, 0)
  line L1 (-46.7, 0) -> (15, 0)
  line L2 (15, 0) -> (15, 10)
  line L3 (15, 10) -> (-46.7, 10)
  line L4 (15, 10) -> (-46.7, 10)
  line L5 (-46.7, 10) -> (-46.7, 5)
  line L6 (-46.7, 5) -> (15, 5)
  line L7 (15, 5) -> (15, 10)
  constraint horizontal L4
  constraint vertical L5
  constraint horizontal L6
  constraint vertical L7
  constraint midpoint L0 L5.end
  constraint coincident L2.end L3.start
extrude "Extrude83" add sketch "Sketch41" along normal blind 5 contours L0 L2 L3 L4 L5 L6 L7 bodies 1
extrude "Extrude84" cut 1 faces at (5.9, 3.3333, 203) along direction (0, 0, -1) blind 5 on bodies 1 bodies 1
extrude "Extrude85" cut 1 faces at (5.9, 8.3333, 208) along direction (0, 0, -1) blind 5 on bodies 1 bodies 1
sketch "Sketch42" plane through (0, 10, 0) normal (0, 1, 0) x (-1, 0, 0)
  line L0 (-47.7, 203) -> (-47.7, 218)
  line L1 (-47.7, 218) -> (-127.2, 218)
  line L2 (-127.2, 218) -> (-127.2, -25)
  line L3 (-127.2, -25) -> (-46.7, -25)
  line L4 (-46.7, -25) -> (-46.7, -10)
  line L5 (-46.7, -10) -> (15, -10)
  line L6 (15, -10) -> (15, 203)
  line L7 (15, 203) -> (-47.7, 203)
  circle A0 centre (-63.325, 91) radius 4
  circle A1 centre (-105.075, 102) radius 4
  line L8 (15, -10) -> (30, -10)
  line L9 (30, -10) -> (30, 203)
  line L10 (30, 203) -> (15, 203)
  line L11 (15, 203) -> (15, -10)
  line L12 (30, 203) -> (15, 203)
  line L13 (15, 203) -> (15, 208)
  line L14 (15, 208) -> (30, 208)
  line L15 (30, 208) -> (30, 203)
  line L16 (15, -10) -> (30, -10)
  line L17 (30, -10) -> (30, -15)
  line L18 (30, -15) -> (15, -15)
  line L19 (15, -15) -> (15, -10)
  line L20 (15, 208) -> (17.475, 208)
  line L21 (17.475, 208) -> (17.475, 203)
  line L22 (17.475, 203) -> (15, 203)
  line L23 (15, 203) -> (15, 208)
  line L24 (15, 208) -> (30, 208)
  line L25 (30, 208) -> (30, 184.5)
  line L26 (30, 184.5) -> (15, 184.5)
  line L27 (15, 184.5) -> (15, 208)
  line L28 (30, 184.5) -> (15, 184.5)
  line L29 (15, 184.5) -> (15, 198)
  line L30 (15, 198) -> (30, 198)
  line L31 (30, 198) -> (30, 184.5)
  line L32 (30, 198) -> (17.475, 208)
  dimension "d243" = 15
  dimension "d244" = 5
  dimension "d245" = 5
  dimension "d246" = 2.475
  dimension "d247" = 23.5
  dimension "d248" = 13.5
  constraint horizontal L8
  constraint vertical L9
  constraint horizontal L10
  constraint vertical L11
  constraint coincident L5.end L6.start
  constraint horizontal L12
  constraint vertical L13
  constraint horizontal L14
  constraint vertical L15
  constraint horizontal L16
  constraint vertical L17
  constraint horizontal L18
  constraint vertical L19
  constraint horizontal L20
  constraint vertical L21
  constraint horizontal L22
  constraint vertical L23
  constraint horizontal L24
  constraint vertical L25
  constraint horizontal L26
  constraint vertical L27
  constraint horizontal L28
  constraint vertical L29
  constraint horizontal L30
  constraint vertical L31
  measures "d243" distance of L5.end L8.end
  measures "d244" distance of L9.end L14.end
  measures "d245" distance of L5.end L18.end
  measures "d246" distance of L13.end L20.end
  measures "d247" distance of L13.end L26.end
  measures "d248" distance of L25.end L30.end
extrude "Extrude86" add sketch "Sketch42" against normal blind 5 contours L6 L10 L11 L12 L22 L27 L30 L32 | L10 L12 L13 L14 L20 L21 L22 L23 L24 L27 | L6 L9 L11 L25 L26 L27 L28 L29 L30 L31 | L10 L12 L21 L32 | L6 L8 L9 L11 L16 L26 L28 | L8 L16 L17 L18 L19 bodies 1